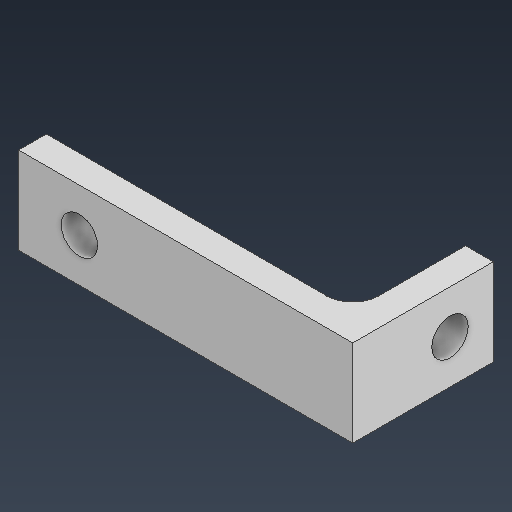
# Autodesk Inventor part: мертвое колесо крепл 2 25-26
Saved by Autodesk Inventor 2025 (Build 290162000, 162)
## iProperties
Created: 2025-09-25
Part Number: мертвое колесо крепл 2 25-26
Material: Типовые
Document SubType Name: Modeling
Designer: GameHD
Density: 1 g/cm^3
Appearance: По умолчанию
Author: GameHD
Autodesk Inventor part; units mm, degrees
ref_plane "YZ Plane" through (0, 0, 0) normal (1, 0, 0) x (0, 1, 0)
ref_plane "XZ Plane" through (0, 0, 0) normal (0, 1, 0) x (-1, 0, 0)
ref_plane "XY Plane" through (0, 0, 0) normal (0, 0, 1) x (1, 0, 0)
sketch "Эскиз1" plane through (0, 0, 0) normal (0, 0, 1) x (1, 0, 0)
  circle A0 centre (0, 0) radius 2.1
  line L0 (-31.5, -5) -> (31.5, -5)
  line L1 (31.5, -5) -> (31.5, 5)
  line L2 (31.5, 5) -> (-31.5, 5)
  line L3 (-31.5, 5) -> (-31.5, -5)
  line L4 (-31.5, -5) -> (31.5, 5) construction
  line L5 (31.5, -5) -> (-31.5, 5) construction
  line L6 (-7, 5) -> (-7, -5)
  dimension "d0" = 4.2
  dimension "d1" = 63
  dimension "d2" = 10
  dimension "d3" = 7
  constraints: 14 end point, 2 midpoint, 2 parallel, 2 perpendicular, 2 point on line, 1 centre point, 1 coincident, 1 horizontal
  measures "d0" diameter of A0
  measures "d1" distance of L2.end L1.end
  measures "d2" distance of L1.end L0.end
  measures "d3" distance from line of point (0, 0) L6
extrude "Выдавливание1" add sketch "Эскиз1" along normal blind 3.2 contours L6 L2 L1 L0
sketch "Эскиз2" plane through (0, 0, 0) normal (0, 0, -1) x (-1, 0, 0)
  line L0 (-31.5, 5) -> (7, 5) projected
  line L1 (7, -5) -> (-31.5, -5) projected
  line L2 (-31.5, 5) -> (-28.3, 5)
  line L3 (-28.3, 5) -> (-28.3, -5)
  line L4 (-28.3, -5) -> (-31.5, -5)
  line L5 (-31.5, -5) -> (-31.5, 5)
  point P0 (0, 0)
  point P1 (-28.3, 5)
  dimension "d6" = 3.2
  constraints: 8 end point, 2 parallel, 1 horizontal, 1 perpendicular, 1 point on line
  measures "d6" distance of L3.end L4.end
extrude "Выдавливание2" add sketch "Эскиз2" along normal blind 13
fillet "Сопряжение1" radius 3 1 edges at (28.3, 0, 0)
sketch "Эскиз3" plane through (28.3, -5, -13) normal (-1, 0, 0) x (0, 0, 1)
  line L0 (0, 0) -> (0, 10) projected
  line L1 (0, 5) -> (10, 5)
  line L2 (10, 10) -> (10, 0) projected
  circle A0 centre (5, 5) radius 2.1
  point P0 (13, 5)
  dimension "d10" = 4.2
  constraints: 3 midpoint, 2 end point, 1 centre point
  measures "d10" diameter of A0
extrude "Выдавливание3" cut sketch "Эскиз3" against normal blind 13
